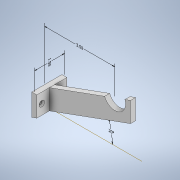
# Autodesk Inventor part: PipeSupport-3_5--020
Saved by Autodesk Inventor 2021.1 (Build 251245010, 245A)
## iProperties
Created: 2020-09-15
Part Number: PipeSupport-3_5--020
Material: Generic
Document SubType Name: Modeling
Designer: robst
Density: 1 g/cm^3
Appearance: Default
Author: robst
Autodesk Inventor part; units mm, degrees
ref_plane "YZ Plane" through (0, 0, 0) normal (1, 0, 0) x (0, 1, 0)
ref_plane "XZ Plane" through (0, 0, 0) normal (0, 1, 0) x (-1, 0, 0)
ref_plane "XY Plane" through (0, 0, 0) normal (0, 0, 1) x (1, 0, 0)
sketch "Sketch5" plane through (0, 0, 0) normal (0, 0, 1) x (1, 0, 0)
  line L0 (0, 0) -> (6.35, 0)
  line L1 (6.35, 0) -> (6.35, 25.4)
  line L2 (6.35, 25.4) -> (0, 25.4)
  line L3 (0, 25.4) -> (0, 0)
  dimension "d21" = 25.4
  dimension "d22" = 6.35
  constraints: 8 end point, 2 parallel, 1 horizontal, 1 perpendicular
  measures "d21" distance from line of L2 L0.start
  measures "d22" distance from line of L1 L0.start
extrude "Extrusion3" add sketch "Sketch5" against normal mid plane 38.1
sketch "Sketch6" plane through (0, 0, 0) normal (0, 0, 1) x (1, 0, 0)
  line L0 (6.35, 25.4) -> (6.35, 0) projected
  line L1 (0, 25.4) -> (6.35, 25.4) projected
  line L2 (6.35, 0) -> (0, 0) projected
  line L3 (0, 0) -> (0, 25.4) projected
  line L4 (6.35, 0) -> (108.9025, 37.3261)
  line L5 (6.35, 0) -> (115.4841, 0) construction
  line L6 (108.9025, 62.7261) -> (108.9025, 37.3261)
  arc A0 (76.0708, 50.7763) -> (101.7292, 60.1152) centre (88.9, 55.4457) ccw
  line L7 (6.35, 25.4) -> (76.0708, 50.7763)
  line L8 (101.7292, 60.1152) -> (108.9025, 62.7261)
  dimension "d25" = 20
  dimension "d26" = 27.305
  dimension "d29" = 6.35
  dimension "d30" = 88.9
  dimension "d33" = 0
  constraints: 10 end point, 2 parallel, 2 point on circle, 1 centre point, 1 collinear, 1 equal length, 1 horizontal, 1 vertical
  measures "d25" angle of L5 L4
  measures "d26" diameter of A0
  measures "d29" distance edge to line of A0 L6
  measures "d30" distance from line of A0.centre L3
  measures "d33" distance from line of L7 A0.centre
extrude "Extrusion4" add sketch "Sketch6" along normal mid plane 6.35 contours L7 A0 L8 L6 L4 L0
sketch "Sketch7" plane through (6.35, 0, 19.05) normal (1, 0, 0) x (0, 0, -1)
  line L0 (38.1, 25.4) -> (0, 25.4) construction
  line L1 (6.35, 25.4) -> (6.35, 0) construction
  line L2 (31.75, 25.4) -> (31.75, 0) construction
  line L3 (0, 0) -> (0, 25.4) construction
  line L4 (38.1, 25.4) -> (38.1, 0) construction
  line L5 (0, 0) -> (15.875, 0) projected
  line L6 (22.225, 0) -> (38.1, 0) projected
  point P0 (19.05, 0)
  point P1 (6.35, 12.7)
  point P2 (31.75, 12.7)
  dimension "d34" = 6.35
  dimension "d35" = 6.35
  constraints: 4 end point, 2 midpoint, 2 point on line, 2 vertical
  measures "d34" distance between parallel lines of L1 L3
  measures "d35" distance between parallel lines of L2 L4
sketch "Sketch8" plane through (0, 0, 0) normal (0, 0, 1) x (1, 0, 0)
  line L0 (0, 0) -> (0, 25.4) projected
  line L1 (6.35, 0) -> (0, 0) projected
  line L2 (108.9025, 37.3261) -> (6.35, 0) projected
  line L3 (0, 0) -> (6.35, 0)
  line L4 (0, -2.3112) -> (6.35, 0)
  line L5 (0, 0) -> (0, -2.3112)
  constraints: 6 end point, 2 collinear, 1 vertical
extrude "Extrusion5" add sketch "Sketch8" along normal mid plane 38.1
hole "Hole3" at (6.35, 12.7, 12.7) at (6.35, 12.7, -12.7) direction (-1, 0, 0) diameter 3.81 end through all countersink diameter 7.0866 countersink angle 82 clearance for "Flat Head Machine Screw (82)" size "#6" standard "Ansi Unified Screw Threads"
sketch "Sketch9" plane through (0, 25.4, -19.05) normal (-1, 0, 0) x (0, 0, 1)
  line L0 (0, -27.7112) -> (0, 0) projected
  line L1 (38.1, 0) -> (38.1, -27.7112) projected
  line L2 (0, -13.8556) -> (38.1, -13.8556) construction
  spline S0 degree 2 poles (12.4032, -12.6206) (12.292, -12.6206) (12.0722, -12.6749) (11.966, -12.7169) knots 0 0 0 1 2 2 2
  spline S1 degree 2 poles (11.966, -12.7169) (11.8672, -12.7589) (11.7215, -12.8478) (11.6647, -12.8874) knots 0 0 0 1 2 2 2
  line L3 (11.6647, -12.8874) -> (11.64, -12.8874)
  line L4 (11.64, -12.8874) -> (11.64, -12.4551)
  spline S2 degree 2 poles (11.64, -12.4551) (11.7733, -12.3835) (12.2303, -12.2674) (12.4353, -12.2674) knots 0 0 0 1 2 2 2
  spline S3 degree 2 poles (12.4353, -12.2674) (12.6428, -12.2674) (12.9515, -12.3514) (13.0775, -12.4403) knots 0 0 0 1 2 2 2
  spline S4 degree 2 poles (13.0775, -12.4403) (13.2109, -12.5366) (13.3492, -12.8157) (13.3492, -13.0034) knots 0 0 0 1 2 2 2
  spline S5 degree 2 poles (13.3492, -13.0034) (13.3492, -13.2554) (13.0182, -13.6358) (12.786, -13.6852) knots 0 0 0 1 2 2 2
  line L5 (12.786, -13.6852) -> (12.786, -13.7148)
  spline S6 degree 2 poles (12.786, -13.7148) (12.8824, -13.7346) (13.1022, -13.8235) (13.1961, -13.9124) knots 0 0 0 1 2 2 2
  spline S7 degree 2 poles (13.1961, -13.9124) (13.2899, -13.9989) (13.4085, -14.2755) (13.4085, -14.4756) knots 0 0 0 1 2 2 2
  spline S8 degree 2 poles (13.4085, -14.4756) (13.4085, -14.6806) (13.2677, -15.0289) (13.1393, -15.1622) knots 0 0 0 1 2 2 2
  spline S9 degree 2 poles (13.1393, -15.1622) (13.0059, -15.3006) (12.628, -15.4438) (12.3884, -15.4438) knots 0 0 0 1 2 2 2
  spline S10 degree 2 poles (12.3884, -15.4438) (12.1587, -15.4438) (11.7091, -15.3327) (11.556, -15.2561) knots 0 0 0 1 2 2 2
  line L6 (11.556, -15.2561) -> (11.556, -14.8239)
  line L7 (11.556, -14.8239) -> (11.5856, -14.8239)
  spline S11 degree 2 poles (11.5856, -14.8239) (11.7141, -14.9177) (12.1488, -15.0906) (12.3637, -15.0906) knots 0 0 0 1 2 2 2
  spline S12 degree 2 poles (12.3637, -15.0906) (12.4896, -15.0906) (12.7416, -15.0116) (12.8256, -14.9202) knots 0 0 0 1 2 2 2
  spline S13 degree 2 poles (12.8256, -14.9202) (12.9071, -14.8288) (12.9935, -14.6114) (12.9935, -14.4459) knots 0 0 0 1 2 2 2
  spline S14 degree 2 poles (12.9935, -14.4459) (12.9935, -14.2804) (12.8972, -14.0656) (12.8107, -14.0038) knots 0 0 0 1 2 2 2
  spline S15 degree 2 poles (12.8107, -14.0038) (12.7243, -13.9421) (12.4896, -13.8951) (12.3513, -13.8951) knots 0 0 0 1 2 2 2
  line L8 (12.3513, -13.8951) -> (12.1784, -13.8951)
  line L9 (12.1784, -13.8951) -> (12.1784, -13.5567)
  line L10 (12.1784, -13.5567) -> (12.3143, -13.5567)
  spline S16 degree 2 poles (12.3143, -13.5567) (12.5884, -13.5567) (12.9342, -13.2949) (12.9342, -13.0454) knots 0 0 0 1 2 2 2
  spline S17 degree 2 poles (12.9342, -13.0454) (12.9342, -12.9293) (12.8453, -12.7639) (12.7737, -12.7145) knots 0 0 0 1 2 2 2
  spline S18 degree 2 poles (12.7737, -12.7145) (12.6971, -12.6626) (12.5094, -12.6206) (12.4032, -12.6206) knots 0 0 0 1 2 2 2
  line L11 (14.5225, -15.3796) -> (14.0334, -15.3796)
  line L12 (14.0334, -15.3796) -> (14.0334, -14.7967)
  line L13 (14.0334, -14.7967) -> (14.5225, -14.7967)
  line L14 (14.5225, -14.7967) -> (14.5225, -15.3796)
  spline S19 degree 2 poles (16.9851, -14.4114) (16.9851, -14.6312) (16.8443, -15.0066) (16.7158, -15.145) knots 0 0 0 1 2 2 2
  spline S20 degree 2 poles (16.7158, -15.145) (16.5874, -15.2833) (16.2045, -15.4438) (15.9674, -15.4438) knots 0 0 0 1 2 2 2
  spline S21 degree 2 poles (15.9674, -15.4438) (15.7501, -15.4438) (15.3252, -15.3475) (15.1696, -15.2709) knots 0 0 0 1 2 2 2
  line L15 (15.1696, -15.2709) -> (15.1696, -14.8387)
  line L16 (15.1696, -14.8387) -> (15.1992, -14.8387)
  spline S22 degree 2 poles (15.1992, -14.8387) (15.2462, -14.8733) (15.4215, -14.9622) (15.5278, -15.0017) knots 0 0 0 1 2 2 2
  spline S23 degree 2 poles (15.5278, -15.0017) (15.6488, -15.0437) (15.8489, -15.0906) (15.9748, -15.0906) knots 0 0 0 1 2 2 2
  spline S24 degree 2 poles (15.9748, -15.0906) (16.0983, -15.0906) (16.3305, -15.0017) (16.4145, -14.9054) knots 0 0 0 1 2 2 2
  spline S25 degree 2 poles (16.4145, -14.9054) (16.4911, -14.814) (16.5701, -14.5719) (16.5701, -14.4089) knots 0 0 0 1 2 2 2
  spline S26 degree 2 poles (16.5701, -14.4089) (16.5701, -14.2459) (16.4812, -14.0384) (16.3972, -13.9692) knots 0 0 0 1 2 2 2
  spline S27 degree 2 poles (16.3972, -13.9692) (16.3108, -13.8927) (16.0539, -13.8284) (15.8983, -13.8284) knots 0 0 0 1 2 2 2
  spline S28 degree 2 poles (15.8983, -13.8284) (15.7303, -13.8284) (15.3968, -13.8803) (15.2956, -13.9025) knots 0 0 0 1 2 2 2
  line L17 (15.2956, -13.9025) -> (15.2956, -12.3316)
  line L18 (15.2956, -12.3316) -> (16.9678, -12.3316)
  line L19 (16.9678, -12.3316) -> (16.9678, -12.6898)
  line L20 (16.9678, -12.6898) -> (15.6883, -12.6898)
  line L21 (15.6883, -12.6898) -> (15.6883, -13.5024)
  spline S29 degree 2 poles (15.6883, -13.5024) (15.7624, -13.4925) (15.9057, -13.4851) (15.965, -13.4851) knots 0 0 0 1 2 2 2
  spline S30 degree 2 poles (15.965, -13.4851) (16.1996, -13.4851) (16.5232, -13.5617) (16.6714, -13.6753) knots 0 0 0 1 2 2 2
  spline S31 degree 2 poles (16.6714, -13.6753) (16.822, -13.7889) (16.9851, -14.1347) (16.9851, -14.4114) knots 0 0 0 1 2 2 2
  line L22 (17.8817, -12.1958) -> (17.7928, -13.3814)
  line L23 (17.7928, -13.3814) -> (17.5235, -13.3814)
  line L24 (17.5235, -13.3814) -> (17.4346, -12.1958)
  line L25 (17.4346, -12.1958) -> (17.8817, -12.1958)
  line L26 (18.6523, -12.1958) -> (18.5634, -13.3814)
  line L27 (18.5634, -13.3814) -> (18.2942, -13.3814)
  line L28 (18.2942, -13.3814) -> (18.2053, -12.1958)
  line L29 (18.2053, -12.1958) -> (18.6523, -12.1958)
  line L30 (22.2956, -15.3796) -> (20.4159, -15.3796)
  line L31 (20.4159, -15.3796) -> (20.4159, -14.9474)
  spline S32 degree 2 poles (20.4159, -14.9474) (20.6185, -14.7572) (20.9791, -14.4039) (21.152, -14.2138) knots 0 0 0 1 2 2 2
  spline S33 degree 2 poles (21.152, -14.2138) (21.5003, -13.8309) (21.7547, -13.3715) (21.7547, -13.127) knots 0 0 0 1 2 2 2
  spline S34 degree 2 poles (21.7547, -13.127) (21.7547, -12.9985) (21.6756, -12.8058) (21.604, -12.7441) knots 0 0 0 1 2 2 2
  spline S35 degree 2 poles (21.604, -12.7441) (21.5324, -12.6823) (21.3446, -12.6206) (21.231, -12.6206) knots 0 0 0 1 2 2 2
  spline S36 degree 2 poles (21.231, -12.6206) (21.1223, -12.6206) (20.9, -12.6749) (20.7988, -12.7169) knots 0 0 0 1 2 2 2
  spline S37 degree 2 poles (20.7988, -12.7169) (20.7123, -12.7515) (20.5518, -12.8503) (20.5024, -12.8849) knots 0 0 0 1 2 2 2
  line L32 (20.5024, -12.8849) -> (20.4801, -12.8849)
  line L33 (20.4801, -12.8849) -> (20.4801, -12.4502)
  spline S38 degree 2 poles (20.4801, -12.4502) (20.6061, -12.3884) (21.0581, -12.2674) (21.2607, -12.2674) knots 0 0 0 1 2 2 2
  spline S39 degree 2 poles (21.2607, -12.2674) (21.688, -12.2674) (22.1696, -12.7194) (22.1696, -13.1047) knots 0 0 0 1 2 2 2
  spline S40 degree 2 poles (22.1696, -13.1047) (22.1696, -13.285) (22.0857, -13.5864) (22.0115, -13.7148) knots 0 0 0 1 2 2 2
  spline S41 degree 2 poles (22.0115, -13.7148) (21.9374, -13.8482) (21.7226, -14.11) (21.604, -14.236) knots 0 0 0 1 2 2 2
  spline S42 degree 2 poles (21.604, -14.236) (21.4113, -14.4459) (20.9396, -14.8955) (20.7988, -15.0264) knots 0 0 0 1 2 2 2
  line L34 (20.7988, -15.0264) -> (22.2956, -15.0264)
  line L35 (22.2956, -15.0264) -> (22.2956, -15.3796)
  spline S43 degree 2 poles (24.6001, -13.8556) (24.6001, -14.6757) (24.1234, -15.4438) (23.6269, -15.4438) knots 0 0 0 1 2 2 2
  spline S44 degree 2 poles (23.6269, -15.4438) (23.1231, -15.4438) (22.6513, -14.6608) (22.6513, -13.8581) knots 0 0 0 1 2 2 2
  spline S45 degree 2 poles (22.6513, -13.8581) (22.6513, -13.0331) (23.128, -12.2699) (23.6269, -12.2699) knots 0 0 0 1 2 2 2
  spline S46 degree 2 poles (23.6269, -12.2699) (24.1284, -12.2699) (24.6001, -13.0603) (24.6001, -13.8556) knots 0 0 0 1 2 2 2
  spline S47 degree 2 poles (24.0765, -14.7843) (24.1358, -14.6337) (24.1852, -14.1693) (24.1852, -13.8556) knots 0 0 0 1 2 2 2
  spline S48 degree 2 poles (24.1852, -13.8556) (24.1852, -13.5419) (24.1358, -13.08) (24.074, -12.9244) knots 0 0 0 1 2 2 2
  spline S49 degree 2 poles (24.074, -12.9244) (24.0123, -12.7688) (23.7974, -12.6082) (23.6269, -12.6082) knots 0 0 0 1 2 2 2
  spline S50 degree 2 poles (23.6269, -12.6082) (23.4565, -12.6082) (23.2367, -12.7688) (23.1725, -12.9293) knots 0 0 0 1 2 2 2
  spline S51 degree 2 poles (23.1725, -12.9293) (23.1107, -13.085) (23.0662, -13.5592) (23.0662, -13.8581) knots 0 0 0 1 2 2 2
  spline S52 degree 2 poles (23.0662, -13.8581) (23.0662, -14.1792) (23.1058, -14.609) (23.17, -14.7769) knots 0 0 0 1 2 2 2
  spline S53 degree 2 poles (23.17, -14.7769) (23.2293, -14.935) (23.4491, -15.1054) (23.6269, -15.1054) knots 0 0 0 1 2 2 2
  spline S54 degree 2 poles (23.6269, -15.1054) (23.7949, -15.1054) (24.0147, -14.9449) (24.0765, -14.7843) knots 0 0 0 1 2 2 2
  spline S55 degree 2 poles (26.5341, -13.0578) (26.5341, -13.3863) (26.0846, -13.8358) (25.7561, -13.8358) knots 0 0 0 1 2 2 2
  spline S56 degree 2 poles (25.7561, -13.8358) (25.4301, -13.8358) (24.9756, -13.3888) (24.9756, -13.0578) knots 0 0 0 1 2 2 2
  spline S57 degree 2 poles (24.9756, -13.0578) (24.9756, -12.7293) (25.4251, -12.2797) (25.7561, -12.2797) knots 0 0 0 1 2 2 2
  spline S58 degree 2 poles (25.7561, -12.2797) (26.0846, -12.2797) (26.5341, -12.7293) (26.5341, -13.0578) knots 0 0 0 1 2 2 2
  spline S59 degree 2 poles (26.213, -13.0578) (26.213, -12.8602) (25.9512, -12.591) (25.7561, -12.591) knots 0 0 0 1 2 2 2
  spline S60 degree 2 poles (25.7561, -12.591) (25.5585, -12.591) (25.2967, -12.8602) (25.2967, -13.0578) knots 0 0 0 1 2 2 2
  spline S61 degree 2 poles (25.2967, -13.0578) (25.2967, -13.2579) (25.5634, -13.5246) (25.7561, -13.5246) knots 0 0 0 1 2 2 2
  spline S62 degree 2 poles (25.7561, -13.5246) (25.9512, -13.5246) (26.213, -13.2529) (26.213, -13.0578) knots 0 0 0 1 2 2 2
  point P0 (19.05, -25.4)
  constraints: 2 end point, 2 midpoint, 1 horizontal
extrude "Extrusion6" cut sketch "Sketch9" against normal blind 1.27
equation "\"d21\" = supportHeight"
equation "\"d22\" = supportWidth"
equation "\"d23\" = totalScrewHoldWidth"
equation "\"d25\" = supportAngle"
equation "\"d26\" = pipeDiameter"
equation "\"d30\" = distanceFromWallToPipeCenter"
equation "\"d31\" = supportWidth"
equation "\"d47\" = totalScrewHoldWidth"
equation "\"pipeDiameter\" = 27.305"
equation "\"distanceFromWallToPipeCenter\" = 88.9"
equation "\"supportHeight\" = 25.4"
equation "\"supportWidth\" = 6.35"
equation "\"screwHoldDepth\" = 6.35"
equation "\"totalScrewHoldWidth\" = 38.1"
equation "\"screwPositionFromTop\" = 6.35"
equation "\"supportAngle\" = 20deg"
body "Solid1"
body "Solid2"
